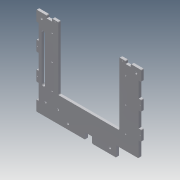
# Autodesk Inventor part: InnerTop
Saved by Autodesk Inventor 2014 (Build 180170000, 170)
## iProperties
Created: 2015-01-19
Part Number: InnerTop
Material: Generic
Document SubType Name: Modeling
Designer: Peele
Density: 1 g/cm^3
Appearance: White
Author: Peele
Autodesk Inventor part; units mm, degrees
ref_plane "YZ Plane" through (0, 0, 0) normal (1, 0, 0) x (0, 1, 0)
ref_plane "XZ Plane" through (0, 0, 0) normal (0, 1, 0) x (-1, 0, 0)
ref_plane "XY Plane" through (0, 0, 0) normal (0, 0, 1) x (1, 0, 0)
sketch "Sketch1" plane through (0, 0, 0) normal (0, 1, 0) x (-1, 0, 0)
  line L0 (125, -92.5) -> (-125, -92.5)
  line L1 (-125, -92.5) -> (-125, 92.5)
  line L2 (-125, 92.5) -> (125, 92.5)
  line L3 (125, 92.5) -> (125, -92.5)
  line L4 (125, -92.5) -> (-125, 92.5) construction
  line L5 (-125, -92.5) -> (125, 92.5) construction
  line L6 (72.5, -57.5) -> (-72.5, -57.5)
  line L7 (-72.5, -57.5) -> (-72.5, 57.5)
  line L8 (-72.5, 57.5) -> (72.5, 57.5)
  line L9 (72.5, 57.5) -> (72.5, -57.5)
  line L10 (72.5, -57.5) -> (-72.5, 57.5) construction
  line L11 (-72.5, -57.5) -> (72.5, 57.5) construction
  line L12 (-90.9745, -29.5734) -> (-84.0255, -29.5734) construction
  line L13 (-84.0255, -29.5734) -> (-84.0255, 29.5734) construction
  line L14 (-84.0255, 29.5734) -> (-90.9745, 29.5734) construction
  line L15 (-90.9745, 29.5734) -> (-90.9745, -29.5734) construction
  line L16 (-90.9745, -29.5734) -> (-84.0255, 29.5734) construction
  line L17 (-84.0255, -29.5734) -> (-90.9745, 29.5734) construction
  line L18 (81.5853, -29.5734) -> (93.4147, -29.5734) construction
  line L19 (93.4147, -29.5734) -> (93.4147, 29.5734) construction
  line L20 (93.4147, 29.5734) -> (81.5853, 29.5734) construction
  line L21 (81.5853, 29.5734) -> (81.5853, -29.5734) construction
  line L22 (81.5853, -29.5734) -> (93.4147, 29.5734) construction
  line L23 (93.4147, -29.5734) -> (81.5853, 29.5734) construction
  point P0 (0, 0)
  point P1 (-87.5, 0)
  point P2 (87.5, 0)
  dimension "d0" = 175
  dimension "d1" = 87.5
  dimension "d2" = 145
  dimension "d4" = 185
  dimension "d5" = 250
  dimension "d15" = 35
  constraints: 48 end point, 8 midpoint, 8 parallel, 4 horizontal, 4 perpendicular
  measures "d0" distance of point (87.5, 0) point (-87.5, 0)
  measures "d1" distance of point (0, 0) point (-87.5, 0)
  measures "d2" distance of L6.start L6.end
  measures "d4" distance of L2.end L0.start
  measures "d5" distance of L0.start L0.end
  measures "d15" distance between parallel lines of L2 L8
extrude "Extrusion1" add sketch "Sketch1" along normal blind 6
sketch "Sketch2" plane through (0, 6, 0) normal (0, 1, 0) x (1, 0, 0)
  line L0 (72.5, -57.5) -> (-72.5, -57.5) projected
  line L1 (-125, -92.5) -> (125, -92.5) projected
  line L2 (-72.5, -57.5) -> (72.5, -57.5)
  line L3 (72.5, -57.5) -> (72.5, -92.5)
  line L4 (72.5, -92.5) -> (-72.5, -92.5)
  line L5 (-72.5, -92.5) -> (-72.5, -57.5)
  point P0 (0, 0)
  constraints: 8 end point, 2 parallel, 1 horizontal, 1 perpendicular, 1 point on line
extrude "Extrusion2" cut sketch "Sketch2" against normal through all
sketch "Sketch3" plane through (0, 0, 0) normal (0, -1, 0) x (1, 0, 0)
  line L0 (-125, 92.5) -> (-125, -92.5) projected
  line L1 (-125, -92.5) -> (125, -92.5) projected
  line L2 (125, -92.5) -> (125, 92.5) projected
  line L3 (-125, -117.5) -> (66, -117.5)
  line L4 (66, -117.5) -> (66, -92.5)
  line L5 (66, -92.5) -> (-125, -92.5)
  line L6 (-125, -92.5) -> (-125, -117.5)
  line L7 (-125, -117.5) -> (66, -92.5) construction
  line L8 (66, -117.5) -> (-125, -92.5) construction
  point P0 (0, 0)
  point P1 (-29.5, -105)
  dimension "d10" = 59
  dimension "d11" = 25
  constraints: 12 end point, 2 midpoint, 2 parallel, 1 collinear, 1 horizontal, 1 perpendicular, 1 point on line
  measures "d10" distance between parallel lines of L2 L4
  measures "d11" distance of L3.end L4.end
extrude "Extrusion3" add sketch "Sketch3" against normal blind 6
sketch "Sketch4" plane through (0, 6, 0) normal (0, 1, 0) x (1, 0, 0)
  line L0 (-72.5, -92.5) -> (-72.5, 57.5) projected
  line L1 (-72.5, 57.5) -> (72.5, 57.5) projected
  line L2 (-125, -92.5) -> (-72.5, -92.5) projected
  line L3 (-108, 53.5) -> (-108, -52.5) construction
  line L4 (-112, 53.5) -> (-112, -52.5)
  line L5 (-104, -52.5) -> (-104, 53.5)
  arc A0 (-104, 53.5) -> (-112, 53.5) centre (-108, 53.5) ccw
  arc A1 (-112, -52.5) -> (-104, -52.5) centre (-108, -52.5) ccw
  point P0 (0, 0)
  point P1 (-108, 0.5)
  dimension "d16" = 8
  dimension "d17" = 108
  dimension "d18" = 40
  constraints: 8 end point, 5 tangent, 4 point on circle, 2 centre point, 2 parallel, 1 midpoint
  measures "d16" distance between parallel lines of L4 L5
  measures "d17" horizontal distance of point (-108, 0.5) point (0, 0)
  measures "d18" distance from line of L3.end L2
extrude "Extrusion4" cut sketch "Sketch4" against normal through all
sketch "Sketch5" plane through (0, 0, 0) normal (0, -1, 0) x (1, 0, 0)
  line L0 (125, 92.5) -> (-125, 92.5) projected
  line L1 (72.5, -57.5) -> (-72.5, -57.5) projected
  circle A0 centre (-87.5, 62.5) radius 1.6
  circle A1 centre (-87.5, 2.5) radius 1.6
  circle A2 centre (-87.5, -57.5) radius 1.6
  circle A3 centre (87.5, 62.5) radius 1.6
  circle A4 centre (87.5, 2.5) radius 1.6
  circle A5 centre (87.5, -57.5) radius 1.6
  line L2 (87.5, 62.5) -> (-87.5, 62.5) construction
  line L3 (0, -57.5) -> (0, 62.5) construction
  line L4 (-95, -72.5) -> (-80, -72.5) construction
  line L5 (-80, -72.5) -> (-80, 77.5) construction
  line L6 (-80, 77.5) -> (-95, 77.5) construction
  line L7 (-95, 77.5) -> (-95, -72.5) construction
  line L8 (-95, -72.5) -> (-80, 77.5) construction
  line L9 (-80, -72.5) -> (-95, 77.5) construction
  point P0 (-72.5, 92.5)
  point P1 (0, 0)
  dimension "d21" = 60
  dimension "d22" = 60
  dimension "d23" = 175
  dimension "d24" = 3.2
  dimension "d25" = 150
  dimension "d26" = 15
  constraints: 16 end point, 6 centre point, 5 equal radius, 4 midpoint, 4 vertical alignment, 3 horizontal alignment, 3 parallel, 1 horizontal, 1 perpendicular, 1 vertical
  measures "d21" distance of L2.start A4.centre
  measures "d22" distance of A5.centre A4.centre
  measures "d23" distance of L2.end L2.start
  measures "d24" diameter of A3
  measures "d25" distance of L6.end L4.start
  measures "d26" distance between parallel lines of L0 L6
extrude "Extrusion5" cut sketch "Sketch5" against normal through all
sketch "Sketch6" plane through (0, 6, 0) normal (0, 1, 0) x (1, 0, 0)
  circle A0 centre (-87.5, 57.5) radius 1.6 projected
  line L0 (66, 117.5) -> (-125, 117.5) projected
  line L1 (-112.5, 60.5) -> (-62.5, 60.5) construction
  line L2 (-62.5, 60.5) -> (-62.5, 114.5) construction
  line L3 (-62.5, 114.5) -> (-112.5, 114.5) construction
  line L4 (-112.5, 114.5) -> (-112.5, 60.5) construction
  line L5 (-112.5, 60.5) -> (-62.5, 114.5) construction
  line L6 (-62.5, 60.5) -> (-112.5, 114.5) construction
  circle A1 centre (-102.5, 87.5) radius 2.2
  circle A2 centre (-72.5, 87.5) radius 2.2
  circle A3 centre (-50, 105) radius 2.7
  circle A4 centre (50, 105) radius 2.7
  line L7 (125, -92.5) -> (125, 92.5) projected
  line L8 (-125, 117.5) -> (-125, -92.5) projected
  line L9 (-125, -92.5) -> (-72.5, -92.5) projected
  circle A5 centre (-112.5, -80) radius 2.7
  circle A6 centre (112.5, -80) radius 2.7
  point P0 (0, 0)
  point P1 (-87.5, 87.5)
  dimension "d29" = 50
  dimension "d30" = 54
  dimension "d31" = 3
  dimension "d32" = 4.4
  dimension "d33" = 30
  dimension "d34" = 15
  dimension "d42" = 12.5
  dimension "d43" = 50
  dimension "d44" = 50
  dimension "d45" = 5.4
  dimension "d46" = 12.5
  dimension "d47" = 12.5
  dimension "d48" = 12.5
  dimension "d49" = 5.4
  dimension "d71" = 12.5
  constraints: 12 end point, 6 centre point, 4 horizontal alignment, 3 equal radius, 2 midpoint, 2 parallel, 1 horizontal, 1 perpendicular, 1 vertical alignment
  measures "d29" distance of L2.end L3.end
  measures "d30" distance of L3.end L1.start
  measures "d31" distance between parallel lines of L0 L3
  measures "d32" diameter of A1
  measures "d33" distance of A1.centre A2.centre
  measures "d34" distance of point (-87.5, 87.5) A2.centre
  measures "d42" distance from line of A4.centre L0
  measures "d43" horizontal distance of A4.centre point (0, 0)
  measures "d44" horizontal distance of A3.centre point (0, 0)
  measures "d45" diameter of A4
  measures "d46" distance from line of A5.centre L8
  measures "d47" distance from line of A5.centre L9
  measures "d48" distance from line of A6.centre L7
  measures "d49" diameter of A6
  measures "d71" distance between parallel lines of L8 L4
extrude "Extrusion6" cut sketch "Sketch6" against normal through all contours A1 | A2 | A3 | A4 | A5 | A6
sketch "Sketch7" plane through (0, 6, 0) normal (0, 1, 0) x (1, 0, 0)
  line L0 (66, 117.5) -> (-125, 117.5) projected
  line L1 (-8, 102.5) -> (8, 102.5)
  line L2 (8, 102.5) -> (8, 117.5)
  line L3 (8, 117.5) -> (-8, 117.5)
  line L4 (-8, 117.5) -> (-8, 102.5)
  line L5 (-8, 102.5) -> (8, 117.5) construction
  line L6 (8, 102.5) -> (-8, 117.5) construction
  point P0 (0, 0)
  point P1 (0, 110)
  dimension "d38" = 16
  dimension "d39" = 15
  constraints: 12 end point, 2 midpoint, 2 parallel, 1 horizontal, 1 perpendicular, 1 point on line, 1 vertical alignment
  measures "d38" distance of L1.start L1.end
  measures "d39" distance of L1.end L2.end
extrude "Extrusion7" cut sketch "Sketch7" against normal through all
sketch "Sketch8" plane through (0, 6, 0) normal (0, 1, 0) x (1, 0, 0)
  line L0 (-125, 117.5) -> (-125, -92.5) projected
  line L1 (72.5, -92.5) -> (125, -92.5) projected
  line L2 (125, -92.5) -> (125, 92.5) projected
  line L3 (125, 92.5) -> (66, 92.5) projected
  line L4 (125, 92.5) -> (118.9, 92.5)
  line L5 (118.9, 92.5) -> (118.9, 55.8333)
  line L6 (118.9, 55.8333) -> (125, 55.8333)
  line L7 (125, 55.8333) -> (125, 92.5)
  line L8 (125, -67.5) -> (118.9, -67.5)
  line L9 (118.9, -67.5) -> (118.9, -30.8333)
  line L10 (118.9, -30.8333) -> (125, -30.8333)
  line L11 (125, -30.8333) -> (125, -67.5)
  line L12 (125, 30.8333) -> (118.9, 30.8333)
  line L13 (118.9, 30.8333) -> (118.9, -5.8333)
  line L14 (118.9, -5.8333) -> (125, -5.8333)
  line L15 (125, -5.8333) -> (125, 30.8333)
  line L16 (-125, 92.5) -> (-118.9, 92.5)
  line L17 (-118.9, 92.5) -> (-118.9, 55.8333)
  line L18 (-118.9, 55.8333) -> (-125, 55.8333)
  line L19 (-125, 55.8333) -> (-125, 92.5)
  line L20 (-125, 30.8333) -> (-118.9, 30.8333)
  line L21 (-118.9, 30.8333) -> (-118.9, -5.8333)
  line L22 (-118.9, -5.8333) -> (-125, -5.8333)
  line L23 (-125, -5.8333) -> (-125, 30.8333)
  line L24 (-125, -67.5) -> (-118.9, -67.5)
  line L25 (-118.9, -67.5) -> (-118.9, -30.8333)
  line L26 (-118.9, -30.8333) -> (-125, -30.8333)
  line L27 (-125, -30.8333) -> (-125, -67.5)
  circle A0 centre (121.95, 43.3333) radius 1.1
  circle A1 centre (121.95, -18.3333) radius 1.1
  circle A2 centre (-121.95, -18.3333) radius 1.1
  circle A3 centre (-121.95, 43.3333) radius 1.1
  line L28 (121.95, 55.8333) -> (121.95, 43.3333) construction
  line L29 (-121.95, 55.8333) -> (-121.95, 43.3333) construction
  point P0 (0, 0)
  dimension "d50" = 25
  dimension "d51" = 6.1
  dimension "d52" = 25
  dimension "d53" = 25
  dimension "d54" = 2.2
  dimension "d55" = 12.5
  dimension "d56" = 12.5
  constraints: 52 end point, 13 parallel, 10 equal length, 6 collinear, 6 horizontal, 6 perpendicular, 5 point on line, 4 centre point, 3 equal radius, 2 horizontal alignment, 2 midpoint, 2 vertical alignment, 1 vertical
  measures "d50" distance between parallel lines of L8 L1
  measures "d51" distance of L8.start L8.end
  measures "d52" distance between parallel lines of L6 L12
  measures "d53" distance between parallel lines of L10 L14
  measures "d54" diameter of A0
  measures "d55" distance of L28.start L28.end
  measures "d56" distance from line of A1.centre L14
extrude "Extrusion8" cut sketch "Sketch8" against normal through all
sketch "Sketch9" plane through (0, 6, 0) normal (0, 1, 0) x (1, 0, 0)
  circle A0 centre (-121.95, -18.3333) radius 1.1 projected
  line L0 (-118.9, -67.5) -> (-125, -67.5) projected
  line L1 (-125, -92.5) -> (-72.5, -92.5) projected
  line L2 (72.5, -92.5) -> (125, -92.5) projected
  line L3 (-100, -92.5) -> (-87.5, -92.5)
  line L4 (-87.5, -92.5) -> (-87.5, -86.4)
  line L5 (-87.5, -86.4) -> (-100, -86.4)
  line L6 (-100, -86.4) -> (-100, -92.5)
  line L7 (100, -92.5) -> (87.5, -92.5)
  line L8 (87.5, -92.5) -> (87.5, -86.4)
  line L9 (87.5, -86.4) -> (100, -86.4)
  line L10 (100, -86.4) -> (100, -92.5)
  circle A1 centre (-80.5, -89.45) radius 1.1
  circle A2 centre (80.5, -89.45) radius 1.1
  line L11 (-80.5, -89.45) -> (-87.5, -89.45) construction
  line L12 (-125, -67.5) -> (-125, -92.5) projected
  line L13 (-72.5, -92.5) -> (-72.5, 57.5) projected
  line L14 (72.5, 57.5) -> (72.5, -92.5) projected
  line L15 (125, -92.5) -> (125, -67.5) projected
  point P0 (0, 0)
  dimension "d60" = 12.5
  dimension "d66" = 25
  dimension "d68" = 8
  dimension "d69" = 8
  dimension "d70" = 25
  constraints: 18 end point, 4 parallel, 3 equal length, 3 horizontal, 2 centre point, 2 equal radius, 2 perpendicular, 2 point on line, 1 horizontal alignment, 1 midpoint
  measures "d60" distance of L4.end L5.end
  measures "d66" distance between parallel lines of L12 L6
  measures "d68" distance from line of L11.start L13
  measures "d69" distance from line of L14 A2.centre
  measures "d70" distance between parallel lines of L15 L10
extrude "Extrusion9" cut sketch "Sketch9" against normal through all contours L6 L5 L4 L1 | L8 L9 L10 L2 | A1 | A2
fillet "Fillet1" radius 2 9 edges at (125, 3, 92.5) (72.5, 3, -57.5) (-125, 3, 92.5) (-72.5, 3, -57.5) (66, 3, -117.5) (-125, 3, -117.5) (8, 3, -117.5) (-8, 3, -117.5) (118.9, 3, -92.5)
fillet "Fillet2" radius 2 15 edges at (125, 3, -55.8333) (125, 3, -30.8333) (125, 3, 5.8333) (125, 3, 30.8333) (125, 3, 67.5) (-125, 3, 67.5) (-125, 3, 30.8333) (-125, 3, 5.8333) (-125, 3, -30.8333) (-125, 3, -55.8333) (-125, 3, -92.5) (-100, 3, 92.5) (-87.5, 3, 92.5) (87.5, 3, 92.5) (100, 3, 92.5)
equation "\"d1\" = 0.5 * d0"
equation "\"d22\" = d21"
equation "\"d34\" = 0.5 * d33"
equation "\"d44\" = d43"
equation "\"d53\" = d52"
equation "\"d55\" = 0.5 * d52"
equation "\"d56\" = d55"
body "Solid1"
